Autodesk Fusion 360 part; units mm, degrees
note: some values were not read from the file. Set by a fixed rule: which sketch regions a step uses.
(part 2 of 2)
sketch "Sketch8" plane through (0, 0, 1.6) normal (0, 0, 1) x (-1, 0, 0)
  circle A0 centre (-209.6445, -19.3084) radius 2
  circle A1 centre (-19.1445, -19.3084) radius 2
  line L0 (-228.695, -0.2577) -> (-228.695, -76.4575)
  line L1 (-228.695, -76.4575) -> (-0.0951, -76.4575)
  line L2 (-0.0951, -76.4575) -> (-0.0951, -0.2577)
  line L3 (-0.0951, -0.2577) -> (-228.695, -0.2577)
  line L4 (-207.119, -16.7831) -> (-207.119, -2.7836)
  line L5 (-207.119, -2.7836) -> (-193.12, -2.7836)
  line L6 (-193.12, -2.7836) -> (-193.12, -16.7831)
  line L7 (-193.12, -16.7831) -> (-207.119, -16.7831)
  line L8 (-78.8197, -21.8336) -> (-78.8197, -35.833)
  line L9 (-78.8197, -35.833) -> (-92.819, -35.833)
  line L10 (-92.819, -35.833) -> (-92.819, -21.8336)
  line L11 (-92.819, -21.8336) -> (-78.8197, -21.8336)
  line L12 (-188.069, -21.8336) -> (-174.07, -21.8336)
  line L13 (-174.07, -21.8336) -> (-174.07, -35.833)
  line L14 (-174.07, -35.833) -> (-188.069, -35.833)
  line L15 (-188.069, -35.833) -> (-188.069, -21.8336)
  line L16 (-169.019, -21.8336) -> (-155.02, -21.8336)
  line L17 (-155.02, -21.8336) -> (-155.02, -35.833)
  line L18 (-155.02, -35.833) -> (-169.019, -35.833)
  line L19 (-169.019, -35.833) -> (-169.019, -21.8336)
  line L20 (-78.8197, -73.9331) -> (-92.819, -73.9331)
  line L21 (-92.819, -73.9331) -> (-92.819, -59.9338)
  line L22 (-92.819, -59.9338) -> (-78.8197, -59.9338)
  line L23 (-78.8197, -59.9338) -> (-78.8197, -73.9331)
  line L24 (-73.769, -21.8336) -> (-59.7697, -21.8336)
  line L25 (-59.7697, -21.8336) -> (-59.7697, -35.833)
  line L26 (-59.7697, -35.833) -> (-73.769, -35.833)
  line L27 (-73.769, -35.833) -> (-73.769, -21.8336)
  line L28 (-54.719, -21.8336) -> (-40.7197, -21.8336)
  line L29 (-40.7197, -21.8336) -> (-40.7197, -35.833)
  line L30 (-40.7197, -35.833) -> (-54.719, -35.833)
  line L31 (-54.719, -35.833) -> (-54.719, -21.8336)
  line L32 (-188.069, -2.7836) -> (-174.07, -2.7836)
  line L33 (-174.07, -2.7836) -> (-174.07, -16.7831)
  line L34 (-174.07, -16.7831) -> (-188.069, -16.7831)
  line L35 (-188.069, -16.7831) -> (-188.069, -2.7836)
  line L36 (-59.7697, -16.7831) -> (-73.769, -16.7831)
  line L37 (-73.769, -16.7831) -> (-73.769, -2.7836)
  line L38 (-73.769, -2.7836) -> (-59.7697, -2.7836)
  line L39 (-59.7697, -2.7836) -> (-59.7697, -16.7831)
  line L40 (-40.7197, -2.7836) -> (-40.7197, -16.7831)
  line L41 (-40.7197, -16.7831) -> (-54.719, -16.7831)
  line L42 (-54.719, -16.7831) -> (-54.719, -2.7836)
  line L43 (-54.719, -2.7836) -> (-40.7197, -2.7836)
  line L44 (-135.97, -16.7831) -> (-149.969, -16.7831)
  line L45 (-149.969, -16.7831) -> (-149.969, -2.7836)
  line L46 (-149.969, -2.7836) -> (-135.97, -2.7836)
  line L47 (-135.97, -2.7836) -> (-135.97, -16.7831)
  line L48 (-92.819, -2.7836) -> (-78.8197, -2.7836)
  line L49 (-78.8197, -2.7836) -> (-78.8197, -16.7831)
  line L50 (-78.8197, -16.7831) -> (-92.819, -16.7831)
  line L51 (-92.819, -16.7831) -> (-92.819, -2.7836)
  line L52 (-105.869, -7.4827) -> (-105.869, -3.0138)
  line L53 (-105.869, -3.0138) -> (-104.144, -3.0138)
  line L54 (-104.144, -3.0138) -> (-104.144, -1.8135)
  line L55 (-104.144, -1.8135) -> (-100.845, -1.8135)
  line L56 (-100.845, -1.8135) -> (-100.845, -3.0138)
  line L57 (-100.845, -3.0138) -> (-99.1182, -3.0138)
  line L58 (-99.1182, -3.0138) -> (-99.1182, -9.2838)
  line L59 (-99.1182, -9.2838) -> (-98.2941, -9.2838)
  line L60 (-98.2941, -9.2838) -> (-98.2941, -12.0826)
  line L61 (-98.2941, -12.0826) -> (-99.1182, -12.0826)
  line L62 (-99.1182, -12.0826) -> (-99.1182, -15.3128)
  line L63 (-99.1182, -15.3128) -> (-105.869, -15.3128)
  line L64 (-105.869, -15.3128) -> (-105.869, -12.0826)
  line L65 (-105.869, -12.0826) -> (-107.395, -12.0826)
  line L66 (-107.395, -12.0826) -> (-107.395, -16.7831)
  line L67 (-107.395, -16.7831) -> (-121.394, -16.7831)
  line L68 (-121.394, -16.7831) -> (-121.394, -12.0826)
  line L69 (-121.394, -12.0826) -> (-122.92, -12.0826)
  line L70 (-122.92, -12.0826) -> (-122.92, -15.3128)
  line L71 (-122.92, -15.3128) -> (-129.669, -15.3128)
  line L72 (-129.669, -15.3128) -> (-129.669, -12.0826)
  line L73 (-129.669, -12.0826) -> (-130.495, -12.0826)
  line L74 (-130.495, -12.0826) -> (-130.495, -9.2838)
  line L75 (-130.495, -9.2838) -> (-129.669, -9.2838)
  line L76 (-129.669, -9.2838) -> (-129.669, -3.0138)
  line L77 (-129.669, -3.0138) -> (-127.944, -3.0138)
  line L78 (-127.944, -3.0138) -> (-127.944, -1.8135)
  line L79 (-127.944, -1.8135) -> (-124.645, -1.8135)
  line L80 (-124.645, -1.8135) -> (-124.645, -3.0138)
  line L81 (-124.645, -3.0138) -> (-122.92, -3.0138)
  line L82 (-122.92, -3.0138) -> (-122.92, -7.4827)
  line L83 (-122.92, -7.4827) -> (-121.394, -7.4827)
  line L84 (-121.394, -7.4827) -> (-121.394, -2.7836)
  line L85 (-121.394, -2.7836) -> (-107.395, -2.7836)
  line L86 (-107.395, -2.7836) -> (-107.395, -7.4827)
  line L87 (-107.395, -7.4827) -> (-105.869, -7.4827)
  line L88 (-155.02, -16.7831) -> (-169.019, -16.7831)
  line L89 (-169.019, -16.7831) -> (-169.019, -2.7836)
  line L90 (-169.019, -2.7836) -> (-155.02, -2.7836)
  line L91 (-155.02, -2.7836) -> (-155.02, -16.7831)
  line L92 (-193.12, -21.8336) -> (-193.12, -35.833)
  line L93 (-193.12, -35.833) -> (-207.119, -35.833)
  line L94 (-207.119, -35.833) -> (-207.119, -21.8336)
  line L95 (-207.119, -21.8336) -> (-193.12, -21.8336)
  line L96 (-226.169, -21.8336) -> (-212.17, -21.8336)
  line L97 (-212.17, -21.8336) -> (-212.17, -35.833)
  line L98 (-212.17, -35.833) -> (-226.169, -35.833)
  line L99 (-226.169, -35.833) -> (-226.169, -21.8336)
  line L100 (-212.17, -16.7831) -> (-226.169, -16.7831)
  line L101 (-226.169, -16.7831) -> (-226.169, -2.7836)
  line L102 (-226.169, -2.7836) -> (-212.17, -2.7836)
  line L103 (-212.17, -2.7836) -> (-212.17, -16.7831)
  line L104 (-97.8683, -40.8838) -> (-97.8683, -54.8831)
  line L105 (-97.8683, -54.8831) -> (-111.869, -54.8831)
  line L106 (-111.869, -54.8831) -> (-111.869, -40.8838)
  line L107 (-111.869, -40.8838) -> (-97.8683, -40.8838)
  line L108 (-116.918, -40.8838) -> (-116.918, -54.8831)
  line L109 (-116.918, -54.8831) -> (-130.919, -54.8831)
  line L110 (-130.919, -54.8831) -> (-130.919, -40.8838)
  line L111 (-130.919, -40.8838) -> (-116.918, -40.8838)
  line L112 (-130.919, -35.833) -> (-130.919, -21.8336)
  line L113 (-130.919, -21.8336) -> (-116.918, -21.8336)
  line L114 (-116.918, -21.8336) -> (-116.918, -35.833)
  line L115 (-116.918, -35.833) -> (-130.919, -35.833)
  line L116 (-111.869, -21.8336) -> (-97.8683, -21.8336)
  line L117 (-97.8683, -21.8336) -> (-97.8683, -35.833)
  line L118 (-97.8683, -35.833) -> (-111.869, -35.833)
  line L119 (-111.869, -35.833) -> (-111.869, -21.8336)
  line L120 (-2.6197, -35.833) -> (-16.6192, -35.833)
  line L121 (-16.6192, -35.833) -> (-16.6192, -21.8336)
  line L122 (-16.6192, -21.8336) -> (-2.6197, -21.8336)
  line L123 (-2.6197, -21.8336) -> (-2.6197, -35.833)
  line L124 (-35.669, -21.8336) -> (-21.6697, -21.8336)
  line L125 (-21.6697, -21.8336) -> (-21.6697, -35.833)
  line L126 (-21.6697, -35.833) -> (-35.669, -35.833)
  line L127 (-35.669, -35.833) -> (-35.669, -21.8336)
  line L128 (-35.669, -2.7836) -> (-21.6697, -2.7836)
  line L129 (-21.6697, -2.7836) -> (-21.6697, -16.7831)
  line L130 (-21.6697, -16.7831) -> (-35.669, -16.7831)
  line L131 (-35.669, -16.7831) -> (-35.669, -2.7836)
  line L132 (-2.6197, -16.7831) -> (-16.6192, -16.7831)
  line L133 (-16.6192, -16.7831) -> (-16.6192, -2.7836)
  line L134 (-16.6192, -2.7836) -> (-2.6197, -2.7836)
  line L135 (-2.6197, -2.7836) -> (-2.6197, -16.7831)
  line L136 (-188.069, -54.8831) -> (-188.069, -40.8838)
  line L137 (-188.069, -40.8838) -> (-174.07, -40.8838)
  line L138 (-174.07, -40.8838) -> (-174.07, -54.8831)
  line L139 (-174.07, -54.8831) -> (-188.069, -54.8831)
  line L140 (-174.07, -59.9338) -> (-174.07, -73.9331)
  line L141 (-174.07, -73.9331) -> (-188.069, -73.9331)
  line L142 (-188.069, -73.9331) -> (-188.069, -59.9338)
  line L143 (-188.069, -59.9338) -> (-174.07, -59.9338)
  line L144 (-193.12, -73.9331) -> (-207.119, -73.9331)
  line L145 (-207.119, -73.9331) -> (-207.119, -59.9338)
  line L146 (-207.119, -59.9338) -> (-193.12, -59.9338)
  line L147 (-193.12, -59.9338) -> (-193.12, -73.9331)
  line L148 (-193.12, -54.8831) -> (-207.119, -54.8831)
  line L149 (-207.119, -54.8831) -> (-207.119, -40.8838)
  line L150 (-207.119, -40.8838) -> (-193.12, -40.8838)
  line L151 (-193.12, -40.8838) -> (-193.12, -54.8831)
  line L152 (-21.6697, -40.8838) -> (-21.6697, -54.8831)
  line L153 (-21.6697, -54.8831) -> (-35.669, -54.8831)
  line L154 (-35.669, -54.8831) -> (-35.669, -40.8838)
  line L155 (-35.669, -40.8838) -> (-21.6697, -40.8838)
  line L156 (-21.6697, -73.9331) -> (-35.669, -73.9331)
  line L157 (-35.669, -73.9331) -> (-35.669, -59.9338)
  line L158 (-35.669, -59.9338) -> (-21.6697, -59.9338)
  line L159 (-21.6697, -59.9338) -> (-21.6697, -73.9331)
  line L160 (-40.7197, -73.9331) -> (-54.719, -73.9331)
  line L161 (-54.719, -73.9331) -> (-54.719, -59.9338)
  line L162 (-54.719, -59.9338) -> (-40.7197, -59.9338)
  line L163 (-40.7197, -59.9338) -> (-40.7197, -73.9331)
  line L164 (-54.719, -54.8831) -> (-54.719, -40.8838)
  line L165 (-54.719, -40.8838) -> (-40.7197, -40.8838)
  line L166 (-40.7197, -40.8838) -> (-40.7197, -54.8831)
  line L167 (-40.7197, -54.8831) -> (-54.719, -54.8831)
  line L168 (-226.169, -73.9331) -> (-226.169, -59.9338)
  line L169 (-226.169, -59.9338) -> (-212.17, -59.9338)
  line L170 (-212.17, -59.9338) -> (-212.17, -73.9331)
  line L171 (-212.17, -73.9331) -> (-226.169, -73.9331)
  line L172 (-155.02, -59.9338) -> (-155.02, -73.9331)
  line L173 (-155.02, -73.9331) -> (-169.019, -73.9331)
  line L174 (-169.019, -73.9331) -> (-169.019, -59.9338)
  line L175 (-169.019, -59.9338) -> (-155.02, -59.9338)
  line L176 (-169.019, -54.8831) -> (-169.019, -40.8838)
  line L177 (-169.019, -40.8838) -> (-155.02, -40.8838)
  line L178 (-155.02, -40.8838) -> (-155.02, -54.8831)
  line L179 (-155.02, -54.8831) -> (-169.019, -54.8831)
  line L180 (-73.769, -59.9338) -> (-59.7697, -59.9338)
  line L181 (-59.7697, -59.9338) -> (-59.7697, -73.9331)
  line L182 (-59.7697, -73.9331) -> (-73.769, -73.9331)
  line L183 (-73.769, -73.9331) -> (-73.769, -59.9338)
  line L184 (-2.6197, -73.9331) -> (-16.6192, -73.9331)
  line L185 (-16.6192, -73.9331) -> (-16.6192, -59.9338)
  line L186 (-16.6192, -59.9338) -> (-2.6197, -59.9338)
  line L187 (-2.6197, -59.9338) -> (-2.6197, -73.9331)
  line L188 (-92.819, -40.8838) -> (-78.8197, -40.8838)
  line L189 (-78.8197, -40.8838) -> (-78.8197, -54.8831)
  line L190 (-78.8197, -54.8831) -> (-92.819, -54.8831)
  line L191 (-92.819, -54.8831) -> (-92.819, -40.8838)
  line L192 (-212.17, -54.8831) -> (-226.169, -54.8831)
  line L193 (-226.169, -54.8831) -> (-226.169, -40.8838)
  line L194 (-226.169, -40.8838) -> (-212.17, -40.8838)
  line L195 (-212.17, -40.8838) -> (-212.17, -54.8831)
  line L196 (-116.918, -59.9338) -> (-116.918, -73.9331)
  line L197 (-116.918, -73.9331) -> (-130.919, -73.9331)
  line L198 (-130.919, -73.9331) -> (-130.919, -59.9338)
  line L199 (-130.919, -59.9338) -> (-116.918, -59.9338)
  line L200 (-135.97, -59.9338) -> (-135.97, -73.9331)
  line L201 (-135.97, -73.9331) -> (-149.969, -73.9331)
  line L202 (-149.969, -73.9331) -> (-149.969, -59.9338)
  line L203 (-149.969, -59.9338) -> (-135.97, -59.9338)
  line L204 (-16.6192, -40.8838) -> (-2.6197, -40.8838)
  line L205 (-2.6197, -40.8838) -> (-2.6197, -54.8831)
  line L206 (-2.6197, -54.8831) -> (-16.6192, -54.8831)
  line L207 (-16.6192, -54.8831) -> (-16.6192, -40.8838)
  line L208 (-135.97, -54.8831) -> (-149.969, -54.8831)
  line L209 (-149.969, -54.8831) -> (-149.969, -40.8838)
  line L210 (-149.969, -40.8838) -> (-135.97, -40.8838)
  line L211 (-135.97, -40.8838) -> (-135.97, -54.8831)
  line L212 (-135.97, -21.8336) -> (-135.97, -35.833)
  line L213 (-135.97, -35.833) -> (-149.969, -35.833)
  line L214 (-149.969, -35.833) -> (-149.969, -21.8336)
  line L215 (-149.969, -21.8336) -> (-135.97, -21.8336)
  line L216 (-73.769, -40.8838) -> (-59.7697, -40.8838)
  line L217 (-59.7697, -40.8838) -> (-59.7697, -54.8831)
  line L218 (-59.7697, -54.8831) -> (-73.769, -54.8831)
  line L219 (-73.769, -54.8831) -> (-73.769, -40.8838)
  line L220 (-111.869, -73.9331) -> (-111.869, -59.9338)
  line L221 (-111.869, -59.9338) -> (-97.8683, -59.9338)
  line L222 (-97.8683, -59.9338) -> (-97.8683, -73.9331)
  line L223 (-97.8683, -73.9331) -> (-111.869, -73.9331)
  circle A2 centre (-38.1944, -57.4085) radius 2
  circle A3 centre (-114.3935, -38.3584) radius 2
  circle A4 centre (-190.5945, -57.4085) radius 2
  line L224 (-0.3951, -76.1575) -> (-228.395, -76.1575)
  line L225 (-228.395, -76.1575) -> (-228.395, -0.5577)
  line L226 (-228.395, -0.5577) -> (-0.3951, -0.5577)
  line L227 (-0.3951, -0.5577) -> (-0.3951, -76.1575)
  dimension "d101" = 0.3
  dimension "d102" = 0.3
  dimension "d103" = 0.3
  dimension "d104" = 0.3
  constraint horizontal L224
  constraint vertical L225
  constraint horizontal L226
  constraint vertical L227
  measures "d101" distance of L1 L224
  measures "d102" distance of L2 L227
  measures "d103" distance of L0 L225
  measures "d104" distance of L3 L226
extrude "Extrude11" cut sketch "Sketch8" against normal blind 15 contours L0 L1 L2 L3 bodies 1
fillet "Fillet7" radius 0.35 4 edges at (0.3951, 0.5577, -0.7) (0.3951, 76.1575, -0.7) (228.395, 0.5577, -0.7) (228.395, 76.1575, -0.7) on bodies 1
sketch "Sketch9" plane through (0, 0, -10) normal (0, 0, 1) x (-1, 0, 0)
  arc A0 (-0.5451, -76.7575) -> (0.2049, -76.0075) centre (-0.5451, -76.0075) ccw
  line L0 (0.2049, -76.0075) -> (0.2049, -0.7077)
  arc A1 (0.2049, -0.7077) -> (-0.5451, 0.0423) centre (-0.5451, -0.7077) ccw
  line L1 (-0.5451, 0.0423) -> (-228.245, 0.0423)
  arc A2 (-228.245, 0.0423) -> (-228.995, -0.7077) centre (-228.245, -0.7077) ccw
  line L2 (-228.995, -0.7077) -> (-228.995, -76.0075)
  arc A3 (-228.995, -76.0075) -> (-228.245, -76.7575) centre (-228.245, -76.0075) ccw
  line L3 (-228.245, -76.7575) -> (-25.1457, -76.7575)
  line L4 (-25.1457, -76.7575) -> (-25.1457, -40)
  line L5 (-25.1457, -40) -> (-1.6912, -40)
  line L6 (-1.6912, -40) -> (-1.6912, -76.7575)
  line L7 (-1.6912, -76.7575) -> (-0.5451, -76.7575)
  circle A4 centre (-209.6445, -19.3084) radius 3.5714
  circle A5 centre (-19.1445, -19.3084) radius 3.5712
  circle A6 centre (-38.1944, -57.4085) radius 3.5714
  circle A7 centre (-114.3935, -38.3584) radius 3.5708
  circle A8 centre (-190.5945, -57.4085) radius 3.5715
  line L8 (-216.0957, -64.0473) -> (-214.8957, -64.0473)
  line L9 (-214.8957, -64.0473) -> (-214.8957, -12.8482)
  line L10 (-214.8957, -12.8482) -> (-216.0957, -12.8482)
  line L11 (-216.0957, -12.8482) -> (-216.0957, -64.0473)
  line L12 (-214.8957, -12.8482) -> (-12.6758, -12.8482)
  line L13 (-12.6758, -12.8482) -> (-12.6758, -14.0482)
  line L14 (-12.6758, -14.0482) -> (-214.8957, -14.0482)
  line L15 (-214.8957, -14.0482) -> (-214.8957, -12.8482)
  line L16 (-12.6758, -14.0482) -> (-13.8758, -14.0482)
  line L17 (-13.8758, -14.0482) -> (-13.8758, -38.7588)
  line L18 (-13.8758, -38.7588) -> (-12.6758, -38.7588)
  line L19 (-12.6758, -38.7588) -> (-12.6758, -14.0482)
  line L20 (-214.8957, -21.2451) -> (-13.4607, -21.2451)
  line L21 (-13.4607, -21.2451) -> (-13.4607, -17.2451)
  line L22 (-13.4607, -17.2451) -> (-214.8957, -17.2451)
  line L23 (-214.8957, -17.2451) -> (-214.8957, -21.2451)
  line L24 (-214.8957, -59.3935) -> (-42.244, -59.3935)
  line L25 (-42.244, -59.3935) -> (-42.244, -55.3935)
  line L26 (-42.244, -55.3935) -> (-214.8957, -55.3935)
  line L27 (-214.8957, -55.3935) -> (-214.8957, -59.3935)
  line L28 (-214.8957, -40.6441) -> (-25.816, -40.6441)
  line L29 (-25.816, -40.6441) -> (-25.816, -36.6441)
  line L30 (-25.816, -36.6441) -> (-214.8957, -36.6441)
  line L31 (-214.8957, -36.6441) -> (-214.8957, -40.6441)
  line L32 (-214.8957, -64.0473) -> (-36.3561, -64.0473)
  line L33 (-36.3561, -64.0473) -> (-36.3561, -62.8473)
  line L34 (-36.3561, -62.8473) -> (-214.8957, -62.8473)
  line L35 (-214.8957, -62.8473) -> (-214.8957, -64.0473)
  circle A9 centre (-38.1944, -57.4085) radius 5
  circle A10 centre (-190.5945, -57.4085) radius 5
  circle A11 centre (-209.6445, -19.3084) radius 5
  circle A12 centre (-114.3935, -38.3584) radius 5
  circle A13 centre (-19.1445, -19.3084) radius 5
  line L36 (-39.6799, -62.1827) -> (-39.6799, -62.8473)
  line L37 (-36.7154, -62.1847) -> (-36.7154, -62.8473)
  line L38 (-192.1228, -62.1692) -> (-192.1228, -62.8473)
  line L39 (-189.0662, -62.1692) -> (-189.0662, -62.8473)
  line L40 (-20.4158, -14.0482) -> (-20.4158, -14.4727)
  line L41 (-17.9485, -14.0482) -> (-17.9485, -14.4535)
  line L42 (-208.4223, -14.0482) -> (-208.4223, -14.46)
  line L43 (-211.0053, -14.0482) -> (-211.0053, -14.4971)
  line L44 (-59.4375, -59.3935) -> (-179.133, -59.3935)
  line L45 (-179.133, -59.3935) -> (-179.133, -58.8935)
  line L46 (-179.133, -58.8935) -> (-59.4375, -58.8935)
  line L47 (-59.4375, -58.8935) -> (-59.4375, -59.3935)
  line L48 (-178.6432, -55.3935) -> (-58.8008, -55.3935)
  line L49 (-58.8008, -55.3935) -> (-58.8008, -55.8935)
  line L50 (-58.8008, -55.8935) -> (-178.6432, -55.8935)
  line L51 (-178.6432, -55.8935) -> (-178.6432, -55.3935)
  line L52 (-125.1542, -40.6441) -> (-204, -40.6441)
  line L53 (-204, -40.6441) -> (-204, -40.1441)
  line L54 (-204, -40.1441) -> (-125.1542, -40.1441)
  line L55 (-125.1542, -40.1441) -> (-125.1542, -40.6441)
  line L56 (-213.7001, -36.6441) -> (-124.7183, -36.6441)
  line L57 (-124.7183, -36.6441) -> (-124.7183, -37.1441)
  line L58 (-124.7183, -37.1441) -> (-213.7001, -37.1441)
  line L59 (-213.7001, -37.1441) -> (-213.7001, -36.6441)
  line L60 (-102.822, -40.6441) -> (-27.915, -40.6441)
  line L61 (-27.915, -40.6441) -> (-27.915, -40.1441)
  line L62 (-27.915, -40.1441) -> (-102.822, -40.1441)
  line L63 (-102.822, -40.1441) -> (-102.822, -40.6441)
  line L64 (-102.6212, -36.6441) -> (-34.0922, -36.6441)
  line L65 (-34.0922, -36.6441) -> (-34.0922, -37.1441)
  line L66 (-34.0922, -37.1441) -> (-102.6212, -37.1441)
  line L67 (-102.6212, -37.1441) -> (-102.6212, -36.6441)
  line L68 (-34.3214, -21.2451) -> (-204.3427, -21.2451)
  line L69 (-204.3427, -21.2451) -> (-204.3427, -20.7451)
  line L70 (-204.3427, -20.7451) -> (-34.3214, -20.7451)
  line L71 (-34.3214, -20.7451) -> (-34.3214, -21.2451)
  line L72 (-24.8557, -17.2451) -> (-204.4211, -17.2451)
  line L73 (-204.4211, -17.2451) -> (-204.4211, -17.7451)
  line L74 (-204.4211, -17.7451) -> (-24.8557, -17.7451)
  line L75 (-24.8557, -17.7451) -> (-24.8557, -17.2451)
  circle A14 centre (-38.1944, -57.4085) radius 3.7
  circle A15 centre (-190.5945, -57.4085) radius 3.7
  circle A16 centre (-209.6445, -19.3084) radius 3.7
  circle A17 centre (-19.1445, -19.3084) radius 3.7
  circle A18 centre (-114.3935, -38.3584) radius 3.7
  line L76 (-48.1263, -55.3935) -> (-51.1263, -55.3935)
  line L77 (-51.1263, -55.3935) -> (-51.1263, -50.3935)
  line L78 (-51.1263, -50.3935) -> (-48.1263, -50.3935)
  line L79 (-48.1263, -50.3935) -> (-48.1263, -55.3935)
  line L80 (-48.1263, -50.3935) -> (-51.1263, -50.3935)
  line L81 (-51.1263, -50.3935) -> (-51.1263, -53.3935)
  line L82 (-51.1263, -53.3935) -> (-48.1263, -53.3935)
  line L83 (-48.1263, -53.3935) -> (-48.1263, -50.3935)
  line L84 (-203.4172, -55.3935) -> (-206.4172, -55.3935)
  line L85 (-206.4172, -55.3935) -> (-206.4172, -50.3935)
  line L86 (-206.4172, -50.3935) -> (-203.4172, -50.3935)
  line L87 (-203.4172, -50.3935) -> (-203.4172, -55.3935)
  line L88 (-203.4172, -50.3935) -> (-206.4172, -50.3935)
  line L89 (-206.4172, -50.3935) -> (-206.4172, -53.3935)
  line L90 (-206.4172, -53.3935) -> (-203.4172, -53.3935)
  line L91 (-203.4172, -53.3935) -> (-203.4172, -50.3935)
  circle A19 centre (-38.1944, -57.4085) radius 5.4388
  circle A20 centre (-38.1944, -57.4085) radius 6.6388
  line L92 (-32.7571, -57.2753) -> (-31.5568, -57.2753)
  line L93 (-32.7571, -57.2753) -> (-33.1961, -57.2753)
  dimension "d107" = 1.2
  dimension "d108" = 1.2
  dimension "d109" = 1.2
  dimension "d110" = 4
  dimension "d111" = 4
  dimension "d112" = 4
  dimension "d113" = 1.2
  dimension "d114" = 10
  dimension "d115" = 10
  dimension "d116" = 10
  dimension "d117" = 10
  dimension "d118" = 10
  dimension "d119" = 0.5
  dimension "d120" = 0.5
  dimension "d121" = 0.5
  dimension "d122" = 0.5
  dimension "d123" = 0.5
  dimension "d124" = 0.5
  dimension "d125" = 0.5
  dimension "d126" = 0.5
  dimension "d127" = 7.4
  dimension "d128" = 7.4
  dimension "d129" = 7.4
  dimension "d130" = 7.4
  dimension "d131" = 7.4
  dimension "d138" = 3
  dimension "d139" = 5
  dimension "d140" = 3
  dimension "d141" = 3
  dimension "d142" = 5
  dimension "d143" = 3
  constraint horizontal L8
  constraint vertical L9
  constraint horizontal L10
  constraint vertical L11
  constraint horizontal L12
  constraint vertical L13
  constraint horizontal L14
  constraint vertical L15
  constraint horizontal L16
  constraint vertical L17
  constraint horizontal L18
  constraint vertical L19
  constraint horizontal L20
  constraint vertical L21
  constraint horizontal L22
  constraint vertical L23
  constraint coincident L9 L20.start
  constraint horizontal L24
  constraint vertical L25
  constraint horizontal L26
  constraint vertical L27
  constraint coincident L9 L24.start
  constraint horizontal L28
  constraint vertical L29
  constraint horizontal L30
  constraint vertical L31
  constraint coincident L9 L28.start
  constraint horizontal L32
  constraint vertical L33
  constraint horizontal L34
  constraint vertical L35
  constraint concentric A6 A9
  constraint concentric A8 A10
  constraint concentric A4 A11
  constraint concentric A7 A12
  constraint concentric A5 A13
  constraint coincident A9 L36.start
  constraint coincident L34 L36.end
  constraint perpendicular L34 L36
  constraint coincident A9 L37.start
  constraint coincident L34 L37.end
  constraint perpendicular L34 L37
  constraint coincident A10 L38.start
  constraint coincident L34 L38.end
  constraint perpendicular L34 L38
  constraint coincident A10 L39.start
  constraint coincident L34 L39.end
  constraint perpendicular L34 L39
  constraint coincident L14 L40.start
  constraint coincident A13 L40.end
  constraint perpendicular L14 L40
  constraint coincident L14 L41.start
  constraint coincident A13 L41.end
  constraint perpendicular L14 L41
  constraint coincident L14 L42.start
  constraint coincident A11 L42.end
  constraint perpendicular L14 L42
  constraint coincident L14 L43.start
  constraint coincident A11 L43.end
  constraint perpendicular L14 L43
  constraint horizontal L44
  constraint vertical L45
  constraint horizontal L46
  constraint vertical L47
  constraint coincident L24 L44.start
  constraint horizontal L48
  constraint vertical L49
  constraint horizontal L50
  constraint vertical L51
  constraint coincident L26 L48.start
  constraint horizontal L52
  constraint vertical L53
  constraint horizontal L54
  constraint vertical L55
  constraint coincident L28 L52.start
  constraint horizontal L56
  constraint vertical L57
  constraint horizontal L58
  constraint vertical L59
  constraint coincident L30 L56.start
  constraint horizontal L60
  constraint vertical L61
  constraint horizontal L62
  constraint vertical L63
  constraint coincident L28 L60.start
  constraint horizontal L64
  constraint vertical L65
  constraint horizontal L66
  constraint vertical L67
  constraint coincident L30 L64.start
  constraint horizontal L68
  constraint vertical L69
  constraint horizontal L70
  constraint vertical L71
  constraint coincident L20 L68.start
  constraint horizontal L72
  constraint vertical L73
  constraint horizontal L74
  constraint vertical L75
  constraint coincident L22 L72.start
  constraint concentric A6 A14
  constraint concentric A8 A15
  constraint concentric A4 A16
  constraint concentric A13 A17
  constraint concentric A12 A18
  constraint horizontal L76
  constraint vertical L77
  constraint horizontal L78
  constraint vertical L79
  constraint coincident L26 L76.start
  constraint horizontal L80
  constraint vertical L81
  constraint horizontal L82
  constraint vertical L83
  constraint horizontal L84
  constraint vertical L85
  constraint horizontal L86
  constraint vertical L87
  constraint coincident L26 L84.start
  constraint horizontal L88
  constraint vertical L89
  constraint horizontal L90
  constraint vertical L91
  constraint concentric A6 A19
  constraint tangent L34 A19
  constraint concentric A9 A20
  constraint tangent L32 A20
  constraint coincident A19 L92.start
  constraint coincident A20 L92.end
  constraint horizontal L92
  constraint coincident A9 L93.end
  constraint parallel L92 L93
  measures "d107" distance of L8.start L8.end
  measures "d108" distance of L9.end L14.end
  measures "d109" distance of L13.end L16.end
  measures "d110" distance of L20.start L22.end
  measures "d111" distance of L24.start L26.end
  measures "d112" distance of L28.start L30.end
  measures "d113" distance of L8.end L34.end
  measures "d114" diameter of A9
  measures "d115" diameter of A10
  measures "d116" diameter of A11
  measures "d117" diameter of A12
  measures "d118" diameter of A13
  measures "d119" distance of L44.start L46.end
  measures "d120" distance of L48.start L50.end
  measures "d121" distance of L52.start L54.end
  measures "d122" distance of L56.start L58.end
  measures "d123" distance of L60.start L62.end
  measures "d124" distance of L64.start L66.end
  measures "d125" distance of L68.start L70.end
  measures "d126" distance of L72.start L74.end
  measures "d127" diameter of A14
  measures "d128" diameter of A15
  measures "d129" diameter of A16
  measures "d130" diameter of A17
  measures "d131" diameter of A18
  measures "d138" distance of L76.start L76.end
  measures "d139" distance of L76.start L78.end
  measures "d140" distance of L78.end L82.end
  measures "d141" distance of L84.start L84.end
  measures "d142" distance of L84.start L86.end
  measures "d143" distance of L86.end L90.end
extrude "Extrude12" add sketch "Sketch9" along normal blind 2.7 separate body contours L22 A11 A16 | L20 L22 A11 A16 | L20 A11 A16 | L20 L22 A11 A16 | L8 L9 L10 L11 L15 L23 L27 L31 L35 | L9 L12 L13 L14 L15 L16 | L22 A13 A17 | L20 L22 A13 A17 | L20 A13 A17 | L20 L22 A13 A17 | L14 L16 L17 L18 L19 L20 L21 L22 | L17 L20 L21 L22 | L30 A12 A18 | L28 L30 A12 A18 | L9 L32 L34 L35 A20 | L24 L26 A10 A15 | L24 A10 A15 | L28 A12 A18 | L28 L30 A12 A18 | L33 L34 A20 | L26 A10 A15 | L33 L34 L37 A19 A20 L92 | L24 L26 A10 A15 | L34 L37 A19 | L24 L25 L26 A9 | L24 L25 L26 A9 makes body 3 at (188.5381, 61.966, -9.1) makes body 4 at (147.8891, 13.2482, -10) makes body 5 at (33.2192, 56.9106, -8.2) makes body 6 at (209.7692, 14.3099, -8.2) makes body 7 at (14.1507, 19.5576, -9.1) makes body 8 at (109.3997, 38.6076, -9.1)
extrude "Extrude13" add sketch "Sketch9" along normal blind 0.4 contours L20 L22 A11 A13 L69 L70 L71 L73 L74 L75 | L9 L20 L22 L23 A11 | L9 L14 L22 A11 L43 | L14 A11 L42 L43 | L14 A13 L40 L41 | L9 L28 L30 L31 A12 L53 L54 L55 L57 L58 L59 | L14 L17 L22 A13 L41 | L17 L20 L22 A13 | L9 L24 L26 L27 A10 L84 | L28 L29 L30 A12 L61 L62 L63 L65 L66 L67 | L34 A10 L38 L39 | L24 L26 A10 L45 L46 L47 L49 L50 L51 L76 A20 | L34 L36 A19 | L24 L26 A19 A20 | L34 L37 A19 | A9 L36 L37 A19 | L24 L26 A9 A19 | A9 L37 A19 L93 bodies 3 4 8 7 5 6
extrude "Extrude14" add sketch "Sketch9" along normal blind 1 contours L22 L72 L73 L74 L75 | L20 L68 L69 L70 L71 | L30 L56 L57 L58 L59 | L28 L52 L53 L54 L55 | L30 L64 L65 L66 L67 | L28 L60 L61 L62 L63 | L26 L48 L49 L50 L51 | L24 L44 L45 L46 L47 bodies 3
fillet "Fillet8" radius 3.5 3 edges at (13.8758, 14.0482, -8.45) (214.8957, 62.8473, -8.65) (214.8957, 14.0482, -8.45) on bodies 3
fillet "Fillet9" radius 4.75 3 edges at (216.0957, 12.8482, -8.65) (12.6758, 12.8482, -8.65) (216.0957, 64.0473, -8.65) on bodies 3
fillet "Fillet10" radius 4 14 edges at (109.6966, 36.6441, -9.8) (119.0904, 36.6441, -9.8) (118.8405, 40.6441, -9.8) (109.9465, 40.6441, -9.8) (205.0348, 21.2451, -9.8) (205.09, 17.2451, -9.8) (186.0185, 55.3935, -9.8) (186.0054, 59.3935, -9.8) (195.1705, 55.3935, -9.8) (195.1836, 59.3935, -9.8) (23.7541, 21.2451, -9.8) (23.6989, 17.2451, -9.8) (42.7704, 55.3935, -9.8) (42.7834, 59.3935, -9.8) on bodies 3
equation "plate_gap = 0.6 mm"
equation "frame_thickness = 1.8 mm"
equation "d7 = frame_thickness"
equation "d8 = frame_thickness"
equation "d9 = frame_thickness"
equation "d10 = frame_thickness"
equation "d11 = plate_thickness"
equation "d15 = border_height_below_plate + border_height_above_plate + plate_thickness"
equation "d17 = border_height_below_plate"
equation "plate_thickness = 1.6 mm"
equation "border_height_above_plate = 5.4 mm"
equation "border_height_below_plate = 11 mm"
equation "d40 = frame_thickness / 2"
equation "screw_hole_diameter = 2 mm"
equation "d62 = screw_hole_diameter"
equation "d63 = screw_hole_diameter"
equation "d64 = screw_hole_diameter"
equation "d65 = screw_hole_diameter"
equation "d66 = screw_hole_diameter"
equation "switch_hook_width = 1.2 mm"
equation "d83 = switch_hook_width"
equation "d84 = switch_hook_width"
equation "d85 = switch_hook_width"
equation "d87 = switch_hook_width"
equation "d88 = switch_hook_width"
equation "d89 = switch_hook_width"
equation "d90 = switch_hook_width"
equation "d91 = switch_hook_width"
named bodies: "Plate", "Lower shell", "Led guide"
